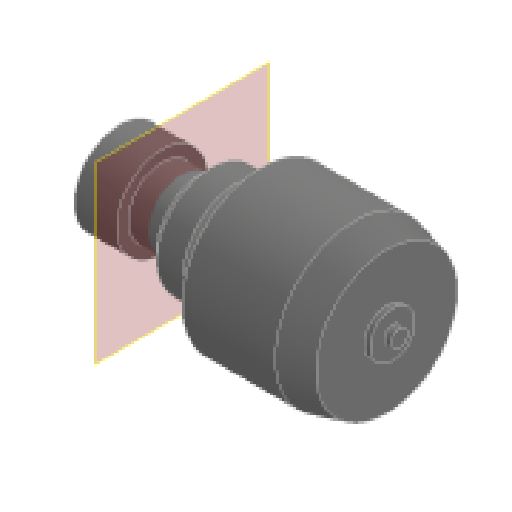
# Autodesk Inventor part: Motor Inverted Pully
Saved by Autodesk Inventor 2023 (Build 270158000, 158)
## iProperties
Created: 2025-02-19
Part Number: Motor Inverted Pully
Material: Generic
Document SubType Name: Modeling
Designer: Ethan
Density: 1 g/cm^3
Appearance: Gray
Author: Ethan
Autodesk Inventor part; units mm, degrees
ref_plane "YZ Plane" through (0, 0, 0) normal (1, 0, 0) x (0, 1, 0)
ref_plane "XZ Plane" through (0, 0, 0) normal (0, 1, 0) x (-1, 0, 0)
ref_plane "XY Plane" through (0, 0, 0) normal (0, 0, 1) x (1, 0, 0)
sketch "Sketch1" plane through (0, 0, 0) normal (0, 1, 0) x (-1, 0, 0)
  line L0 (0, 0) -> (0, -12.5)
  line L1 (0, 0) -> (48.3, 0)
  line L2 (0, -12.5) -> (5.7, -14)
  line L3 (5.7, -14) -> (22.1, -14)
  line L4 (22.1, -14) -> (26.4, -9.5)
  line L5 (26.4, -9.5) -> (31, -9.5)
  line L6 (31, -9.5) -> (31, -3)
  line L7 (31, -3) -> (48.3, -3)
  line L8 (48.3, -3) -> (48.3, 0)
  line L9 (0, -1.5) -> (-2.2, -1.5)
  line L10 (-2.2, -1.5) -> (-2.2, 0)
  line L11 (-2.2, 0) -> (0, 0)
  line L12 (0, 0) -> (0, -4)
  line L13 (0, -4) -> (-1, -4)
  line L14 (-1, -4) -> (-1, -1.5)
  point P0 (0, 0)
  dimension "d2" = 48.3
  dimension "d3" = 9.5
  dimension "d4" = 3
  dimension "d5" = 14
  dimension "d6" = 16.4
  dimension "d7" = 4.6
  dimension "d8" = 31
  dimension "d9" = 5.7
  dimension "d10" = 12.5
  dimension "d19" = 2.2
  dimension "d20" = 1.5
  dimension "d21" = 4
  dimension "d22" = 1
  constraints: 30 end point, 7 perpendicular, 3 horizontal, 3 point on line, 1 coincident, 1 parallel, 1 vertical
  measures "d2" distance of L0.start L1.end
  measures "d3" distance between parallel lines of L1 L5
  measures "d4" distance between parallel lines of L1 L7
  measures "d5" distance between parallel lines of L3 L1
  measures "d6" distance of L2.end L3.end
  measures "d7" distance of L4.end L5.end
  measures "d8" distance between parallel lines of L0 L6
  measures "d9" horizontal distance of L2.end L0.end
  measures "d10" distance of point (0, 0) L0.end
  measures "d19" distance of L9.start L9.end
  measures "d20" distance from line of point (0, 0) L9
  measures "d21" distance of L0.start L12.end
  measures "d22" distance of L12.end L13.end
revolve "Revolution1" add sketch "Sketch1" angle 360 about axis through (0, 0, 0) along (-1, 0, 0)
sketch "Sketch2" plane through (0, 0, 0) normal (0, 1, 0) x (-1, 0, 0)
  line L0 (31, -3) -> (31, 3) projected
  line L1 (31, -9.5) -> (31, 9.5) projected
  line L2 (48.3, -3) -> (48.3, 3) projected
  line L3 (31, -8) -> (32.5, -8)
  line L4 (32.5, -8) -> (32.5, -6)
  line L5 (32.5, -6) -> (39.6, -6)
  line L6 (39.6, -6) -> (39.6, -8)
  line L7 (39.6, -8) -> (47.1, -8)
  line L8 (47.1, -8) -> (47.1, -3)
  line L9 (31, -3) -> (48.3, -3) projected
  line L10 (57.96, 0) -> (-9.66, 0) projected
  point P0 (0, 0)
  dimension "d12" = 1.5
  dimension "d13" = 6
  dimension "d14" = 7.5
  dimension "d15" = 16.1
  dimension "d16" = 8
  dimension "d17" = 8
  constraints: 12 end point, 5 perpendicular, 2 point on line, 1 horizontal
  measures "d12" distance of L3.start L3.end
  measures "d13" distance from line of point (0, 0) L5
  measures "d14" distance of L6.end L7.end
  measures "d15" distance between parallel lines of L1 L8
  measures "d16" distance from line of point (0, 0) L7
  measures "d17" distance from line of point (0, 0) L3
revolve "Revolution2" add sketch "Sketch2" angle 360 about axis through (-10, 0, 0) along (1, 0, 0) contours L9 L8 L7 L6 L5 L4 L3 L1
ref_plane "Work Plane1" through (-36.05, 0, 0) normal (-1, 0, 0) x (0, 0, 1)
body "Solid1"
